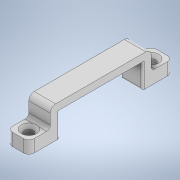
# Autodesk Inventor part: klammern_usbc_hub
Saved by Autodesk Inventor 2021.3 (Build 253353010, 353A)
## iProperties
Created: 2021-07-29
Part Number: klammern_usbc_hub
Material: Generisch
Document SubType Name: Modeling
Designer: Markus
Density: 1 g/cm^3
Appearance: Vorgabe
Author: Markus
Autodesk Inventor part; units mm, degrees
ref_plane "YZ Plane" through (0, 0, 0) normal (1, 0, 0) x (0, 1, 0)
ref_plane "XZ Plane" through (0, 0, 0) normal (0, 1, 0) x (-1, 0, 0)
ref_plane "XY Plane" through (0, 0, 0) normal (0, 0, 1) x (1, 0, 0)
sketch "Skizze1" plane through (0, 0, 0) normal (1, 0, 0) x (0, 1, 0)
  line L0 (13.8, 23.25) -> (13.8, -23.25)
  line L1 (13.8, -23.25) -> (0, -23.25)
  line L2 (0, -23.25) -> (0, -40.25)
  line L3 (0, -40.25) -> (7, -40.25)
  line L4 (7, -40.25) -> (7, -28.25)
  line L5 (7, -28.25) -> (17.8, -28.25)
  line L6 (17.8, -28.25) -> (17.8, 28.25)
  line L7 (17.8, 28.25) -> (7, 28.25)
  line L8 (7, 28.25) -> (7, 40.25)
  line L9 (7, 40.25) -> (0, 40.25)
  line L10 (0, 40.25) -> (0, 23.25)
  line L11 (0, 23.25) -> (13.8, 23.25)
  line L12 (17.8, 0) -> (0, 0) construction
  dimension "d0" = 7
  dimension "d1" = 5
  dimension "d2" = 4
  dimension "d3" = 46.5
  dimension "d4" = 12
  dimension "d12" = 13.8
  constraints: 27 end point, 9 perpendicular, 3 point on line, 1 horizontal, 1 midpoint, 1 parallel, 1 vertical, 1 vertical alignment, 5 other
  measures "d0" distance of L8.end L9.end
  measures "d1" distance between parallel lines of L11 L7
  measures "d2" distance between parallel lines of L6 L0
  measures "d3" distance of L0.start L0.end
  measures "d4" distance of L7.end L8.end
  measures "d12" distance of L0.end L1.end
extrude "Extrusion1" add sketch "Skizze1" along normal blind 12
sketch "Skizze2" plane through (0, 7, 40.25) normal (0, 1, 0) x (1, 0, 0)
  line L0 (0, 12) -> (0, 0) projected
  line L1 (0, 0) -> (12, 0) projected
  line L2 (12, 12) -> (12, 0) projected
  line L3 (0, 12) -> (12, 12) projected
  line L4 (0, 80.5) -> (0, 68.5) projected
  line L5 (0, 68.5) -> (12, 68.5) projected
  line L6 (12, 80.5) -> (12, 68.5) projected
  line L7 (0, 80.5) -> (12, 80.5) projected
  point P0 (0, 40.25)
  point P1 (6, 6)
  point P2 (6, 0)
  point P3 (0, 6)
  point P4 (6, 74.5)
  point P5 (0, 74.5)
  point P6 (6, 80.5)
  constraints: 4 midpoint, 2 horizontal alignment, 2 vertical alignment
hole "Bohrung1" at (6, 7, -34.25) at (6, 7, 34.25) direction (0, -1, 0) diameter 5 end through all countersink diameter 8.6 countersink angle 90
fillet "Rundung1" radius 2 2 edges at (6, 7, 28.25) (6, 7, -28.25)
fillet "Rundung2" radius 3 2 edges at (6, 17.8, 28.25) (6, 17.8, -28.25)
fillet "Rundung3" radius 3 4 edges at (12, 3.5, 40.25) (0, 3.5, 40.25) (12, 3.5, -40.25) (0, 3.5, -40.25)
fillet "Rundung4" radius 1 6 edges at (0, 6.9, 23.25) (12, 6.9, -23.25) (12, 6.9, 23.25) (0, 6.9, -23.25) (6, 0, -23.25) (6, 0, 23.25)
